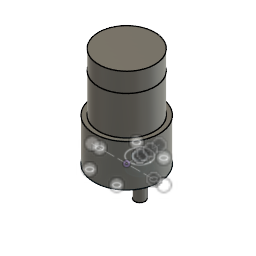
jgb37_520_motor_v0_1 (Autodesk Fusion 360 design; units mm, degrees)
part number: 2026-05-27-19-27-58-394
Autodesk Fusion 360 part; units mm, degrees
cylinder "圆柱体基本要素1" add diameter 37 height 24 placed x (1, 0, 0) y (0, 0, -1) z (0, 1, 0) at (0, 0, 0) makes body 1
cylinder "圆柱体基本要素2" add diameter 32 height 22 placed x (1, 0, 0) y (0, 0, -1) z (0, 1, 0) at (0, 24, 0) bodies 1
cylinder "圆柱体基本要素3" add diameter 32 height 11 placed x (1, 0, 0) y (0, 0, -1) z (0, 1, 0) at (0, 46, 0) separate body makes body 2
sketch "草图5" plane through (0, 0, 0) normal (0, -1, 0) x (1, 0, 0)
  circle A0 centre (0, 0) radius 18.5
  line L0 (0, 0) -> (0, -18.5) construction
  circle A1 centre (0, -7.5) radius 6
  line L1 (1.6583, -10) -> (-1.6583, -10)
  arc A2 (1.6583, -10) -> (-1.6583, -10) centre (0, -7.5) ccw
  circle A3 centre (0, -7.5) radius 3
  circle A4 centre (-15.5, 0) radius 1.6
  circle A5 centre (-7.75, -13.4234) radius 1.6
  circle A6 centre (7.75, -13.4234) radius 1.6
  circle A7 centre (15.5, 0) radius 1.6
  circle A8 centre (7.75, 13.4234) radius 1.6
  circle A9 centre (-7.75, 13.4234) radius 1.6
  line L2 (-19.7514, 0) -> (21.2486, 0) construction
  point P0 (0, -18.5)
  point P1 (0, -7.5)
  point P2 (0, -10)
  point P3 (0, -13.5)
  dimension "d10" = 12
  dimension "d11" = 6
  dimension "d12" = 2.5
  dimension "d13" = 5
  dimension "d20" = 3.2
  dimension "d22" = 360
  dimension "d23" = 31
  constraint coincident A0 P0
  constraint coincident A0.centre L0.start
  constraint coincident P0 L0.end
  constraint coincident L0 P1
  constraint coincident P1 A1.centre
  constraint coincident L0 P2
  constraint perpendicular L0 L1
  constraint coincident P2 L1
  constraint coincident A1 P3
  constraint coincident L0 P3
  constraint concentric A1 A3
  constraint vertical L0
  constraint horizontal L2
  constraint coincident A0.centre L2
  constraint coincident A7.centre L2
  measures "d10" diameter of A1
  measures "d11" diameter of A2
  measures "d12" distance of P1 P2
  measures "d13" distance of P0 P3
  measures "d20" diameter of A4
  measures "d23" distance of A4.centre A7.centre
extrude "拉伸1" add sketch "草图5" along normal blind 6 contours A1 | L1 A3 bodies 1
extrude "拉伸2" add 1 faces at (-0.2173, 0, -8.1906) along direction (0, -1, 0) blind 21 on bodies 1 bodies 1
sketch "草图6" plane through (0, -6, 0) normal (0, -1, 0) x (1, 0, 0)
  arc A0 (1.6583, -10) -> (-1.6583, -10) centre (0, -7.5) ccw
  line L0 (1.6583, -10) -> (-1.6583, -10)
  circle A1 centre (0, -7.5) radius 6
extrude "拉伸3" add sketch "草图5" along normal blind 9 contours L1 A3 | L1 A2 A3 bodies 1
